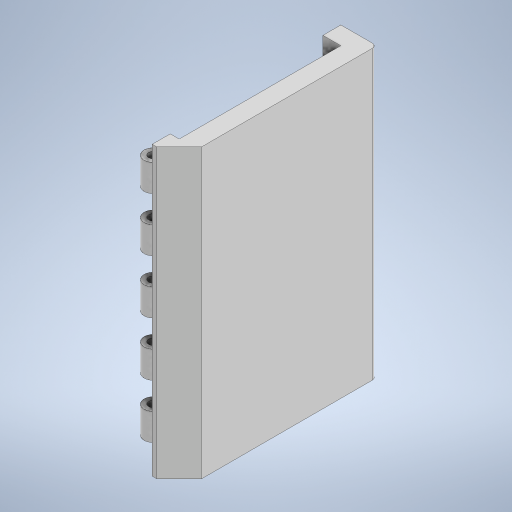
# Autodesk Inventor part: PhoneSafeDoor(H)
Saved by Autodesk Inventor 2023 (Build 270158030, 158C)
## iProperties
Created: 2023-03-04
Part Number: PhoneSafeDoor(H)
Material: Generic
Document SubType Name: Modeling
Designer: mpino
Density: 1 g/cm^3
Appearance: Default
Author: mpino
Autodesk Inventor part; units mm, degrees
ref_plane "YZ Plane" through (0, 0, 0) normal (1, 0, 0) x (0, 1, 0)
ref_plane "XZ Plane" through (0, 0, 0) normal (0, 1, 0) x (-1, 0, 0)
sketch "Sketch1" plane through (0, 0, 0) normal (1, 0, 0) x (0, 1, 0)
  line L0 (0, 0) -> (203.2, 0)
  line L1 (203.2, 0) -> (203.2, -152.4)
  line L2 (203.2, -152.4) -> (0, -152.4)
  line L3 (0, -152.4) -> (0, 0)
  dimension "d0" = 203.2
  dimension "d1" = 152.4
  constraints: 8 end point, 2 parallel, 1 horizontal, 1 perpendicular
  measures "d0" distance of L1.end L2.end
  measures "d1" distance of L0.end L1.end
extrude "Extrusion1" add sketch "Sketch1" along normal blind 12.7
sketch "Sketch2" plane through (0, 0, 0) normal (-1, 0, 0) x (0, 0, 1)
  line L0 (-152.4, 0) -> (-152.4, 203.2) projected
  line L1 (-152.4, 203.2) -> (0, 203.2) projected
  line L2 (-152.4, 0) -> (-139.7, 0)
  line L3 (-139.7, 0) -> (-139.7, 203.2)
  line L4 (-139.7, 203.2) -> (-152.4, 203.2)
  line L5 (-152.4, 203.2) -> (-152.4, 0)
  point P0 (0, 0)
  dimension "d4" = 12.7
  constraints: 8 end point, 2 parallel, 1 horizontal, 1 perpendicular, 1 point on line
  measures "d4" distance of L4.end L3.end
extrude "Extrusion2" add sketch "Sketch2" along normal blind 12.7
fillet "Fillet1" radius 3.175 1 edges at (12.7, 101.6, -152.4)
sketch "Sketch3" plane through (0, 0, 0) normal (0, -1, 0) x (1, 0, 0)
  line L0 (0, 0) -> (0, -12.7)
  line L1 (0, -12.7) -> (0, -25.4)
  line L2 (0, -12.7) -> (-6.35, -12.7)
  line L3 (-6.35, -12.7) -> (-6.35, -25.4)
  line L4 (-6.35, -25.4) -> (0, -25.4)
  dimension "d8" = 12.7
  dimension "d9" = 12.7
  dimension "d10" = 6.35
  dimension "d11" = 90
  constraints: 10 end point, 1 horizontal, 1 parallel, 1 perpendicular, 1 vertical
  measures "d8" distance of L0.start L0.end
  measures "d9" distance of L0.end L1.end
  measures "d10" distance of L0.end L2.end
  measures "d11" angle of L0 L4
extrude "Extrusion3" add sketch "Sketch3" against normal up to surface (203.2 mm away)
ref_plane "Work Plane1" through (0, 19.05, 0) normal (0, -1, 0) x (1, 0, 0)
sketch "Sketch4" plane through (0, 19.05, 0) normal (0, -1, 0) x (1, 0, 0)
  line L0 (0, -19.05) -> (-12.065, -19.05)
  circle A0 centre (-12.065, -19.05) radius 3.175
  circle A1 centre (-12.065, -19.05) radius 6.35
  point P0 (0, 0)
  dimension "d15" = 12.065
  dimension "d16" = 6.35
  dimension "d17" = 12.7
  dimension "d18" = 19.05
  dimension "d19" = 19.05
  constraints: 2 centre point, 2 coincident, 2 end point, 1 horizontal
  measures "d15" distance of L0.start L0.end
  measures "d16" diameter of A0
  measures "d17" diameter of A1
  measures "d18" distance from line of point (0, 0) L0
  measures "d19" distance of point (0, 0) L0.start
extrude "Extrusion4" add sketch "Sketch4" against normal blind 19.05
pattern_linear "Rectangular Pattern1" count 5 spacing 38.1 along (0, 1, 0) of "Extrusion4"
sketch "Sketch5" plane through (0, 203.2, 0) normal (0, 1, 0) x (1, 0, 0)
  line L0 (0, 0) -> (12.7, 0)
  line L1 (12.7, 0) -> (12.7, 12.7)
  line L2 (12.7, 12.7) -> (0, 12.7)
  line L3 (0, 12.7) -> (0, 0)
  line L4 (12.7, 149.225) -> (12.7, 0) projected
  constraints: 8 end point, 2 parallel, 1 coincident, 1 horizontal, 1 perpendicular, 1 point on line
extrude "Extrusion5" cut sketch "Sketch5" against normal blind 203.2
chamfer "Chamfer2" distance 15.875 angle 45 1 edges at (12.7, 101.6, -12.7)
sketch "Sketch6" plane through (-12.7, 0, -152.4) normal (0, 0, -1) x (-1, 0, 0)
  line L0 (0, 0) -> (0, 63.5)
  line L1 (0, 63.5) -> (-6.35, 63.5)
  line L2 (-12.7, 0) -> (-12.7, 203.2) projected
  line L3 (-6.35, 63.5) -> (-12.7, 63.5)
  line L4 (-12.7, 63.5) -> (-12.7, 114.3)
  line L5 (-12.7, 114.3) -> (-6.35, 114.3)
  line L6 (-6.35, 114.3) -> (-6.35, 63.5)
  dimension "d35" = 63.5
  dimension "d37" = 6.35
  dimension "d38" = 50.8
  constraints: 12 end point, 3 parallel, 2 perpendicular, 1 horizontal, 1 point on line
  measures "d35" distance of L0.start L0.end
  measures "d37" distance of L0.end L1.end
  measures "d38" distance of L3.end L4.end
extrude "Extrusion6" cut sketch "Sketch6" against normal blind 3.81
body "Solid1"
